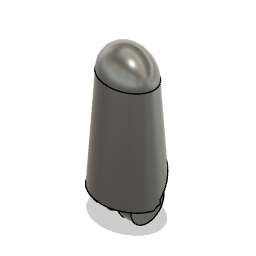
Bionic hand- flextion extention v2 (Autodesk Fusion 360 archive; units mm, degrees)
design "index part 1"
Autodesk Fusion 360 part; units mm, degrees
sketch "1st ellipse" plane through (0, 0, 0) normal (0, 1, 0) x (1, 0, 0)
  ellipse E0 centre (0, 0) end of major axis (5, 0) minor radius 4
  line L0 (-5, 0) -> (5, 0) construction
  line L1 (0, -4) -> (0, 4) construction
  constraint coincident E0 L0.start
  constraint coincident E0 L0.end
  constraint coincident E0 L1.start
  constraint coincident E0 L1.end
  constraint coincident E0.centre origin
  constraint horizontal L0
ref_plane "WorkPlane1" through (0, 15, 0) normal (0, 1, 0) x (1, 0, 0)
sketch "top elipse" plane through (0, 15, 0) normal (0, 1, 0) x (1, 0, 0)
  ellipse E0 centre (0, 0) end of major axis (4, 0) minor radius 3
  line L0 (-4, 0) -> (4, 0) construction
  line L1 (0, -3) -> (0, 3) construction
  constraint coincident E0 L0.start
  constraint coincident E0 L0.end
  constraint coincident E0 L1.start
  constraint coincident E0 L1.end
  constraint coincident E0.centre origin
  constraint horizontal L0
loft "Loft1" add profiles "1st ellipse", "top elipse" section 1 section 2 makes body 1
sketch "line over small elipse" plane through (0, 15, 0) normal (0, 1, 0) x (-1, 0, 0)
  ellipse E0 centre (0, 0) end of major axis (-4, 0) minor radius 3
  ellipse E1 centre (0, 0) end of major axis (-4, 0) minor radius 3
  line L0 (4, 0) -> (-4, 0) construction
  line L1 (0, 3) -> (0, -3) construction
  line L2 (0, -3) -> (0, 3)
  constraint coincident E1 L0.start
  constraint coincident E1 L0.end
  constraint coincident E1 L1.start
  constraint coincident E1 L1.end
  constraint coincident E0.centre E1.centre
  constraint horizontal L0
  constraint coincident L1.end L2.start
  constraint coincident L1.start L2.end
revolve "Revolve1" add sketch "line over small elipse" angle 360 about axis through (0, 15, 3) along (0, 0, -1) separate body contours E0 E1 L2 picked at (-0.4011, 0.9861) makes body 2
sketch "trapezium " plane through (0, 0, 0) normal (1, 0, 0) x (0, 0, -1)
  line L0 (0, 0) -> (0, 1)
  line L1 (0, 1) -> (4.5, 5.5)
  line L2 (4.5, 5.5) -> (4.5, 0)
  line L3 (4.5, 0) -> (0, 0)
  dimension "d3" = 1
  constraint coincident L0.start L3.end
  constraint vertical L0
  constraint parallel L0 L2
  constraint perpendicular L0 L3
  measures "d3" distance of L0.start L0.end
extrude "Extrude1" cut sketch "trapezium " along normal through all and the other way through all bodies 1
sketch "big circle" plane through (0, 0, 0) normal (1, 0, 0) x (0, 0, -1)
  circle A0 centre (0, -0.5) radius 2.5
  dimension "d5" = 5
  measures "d5" diameter of A0
extrude "Extrude2" add sketch "big circle" along normal mid plane 6 separate body makes body 3
extrude "Extrude3" cut 1 faces at (-3, -1.0437, -0.4573) along direction (1, 0, 0) blind 2 on bodies 3 bodies 1 3
extrude "Extrude4" cut 1 faces at (3, -1.0437, -0.4573) along direction (-1, 0, 0) blind 2 on bodies 3 bodies 1 3
sketch "small circle" plane through (-3, 0, 0) normal (1, 0, 0) x (0, 0, -1)
  line L0 (0, 1) -> (0.8508, 1.8508)
  arc A0 (0.8508, 1.8508) -> (-2.4495, 0) centre (0, -0.5) ccw
  line L1 (-2.4495, 0) -> (0, 0)
  line L2 (0, 0) -> (0, 1)
  circle A1 centre (0, -0.5) radius 1
  dimension "d12" = 2
  constraint concentric A0 A1
  measures "d12" diameter of A1
extrude "Extrude5" cut sketch "small circle" along normal mid plane 18 contours L1 L2 A1 | L1 L2 A1 bodies 1 3
sketch "Sketch7" plane through (0, 0, 0) normal (0, 0, 1) x (1, 0, 0)
sketch "Sketch8" plane through (0, 0, 0) normal (1, 0, 0) x (0, 0, -1)
extrude "Extrude6" add 1 faces at (1, -0.6739, -1.987) along direction (1, 0, 0) blind 2 on bodies 3 bodies 1 2 3
extrude "Extrude7" cut 1 faces at (-1, -2.4451, 0.4457) along direction (1, 0, 0) blind 2 on bodies 1 bodies 1
sketch "Sketch9" plane through (0, 0, 0) normal (1, 0, 0) x (0, 0, -1)
  circle A0 centre (0, -0.5) radius 2.5
  dimension "d19" = 5
  measures "d19" diameter of A0
extrude "Extrude8" add sketch "Sketch9" against normal blind 3 separate body makes body 4
extrude "Extrude9" cut 1 faces at (0, 0.1515, -0.5196) along direction (-1, 0, 0) blind 1 on bodies 4 bodies 4
extrude "Extrude10" cut sketch "small circle" along normal blind 3 contours L1 L2 A1 | L1 L2 A1 bodies 4

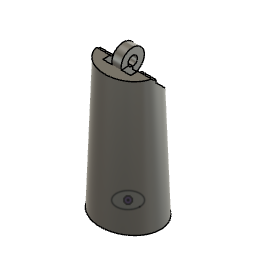
design "middle part 3"
Autodesk Fusion 360 part; units mm, degrees
sketch "Sketch1" plane through (0, 0, 0) normal (0, 1, 0) x (1, 0, 0)
  ellipse E0 centre (0, 0) end of major axis (7, 0) minor radius 6
  line L0 (-7, 0) -> (7, 0) construction
  line L1 (0, -6) -> (0, 6) construction
  dimension "d2" = 12
  constraint coincident E0 L0.start
  constraint coincident E0 L0.end
  constraint coincident E0 L1.start
  constraint coincident E0 L1.end
  constraint coincident E0.centre origin
  constraint horizontal L0
ref_plane "WorkPlane1" through (0, 28, 0) normal (0, 1, 0) x (1, 0, 0)
sketch "Sketch2" plane through (0, 28, 0) normal (0, 1, 0) x (1, 0, 0)
  ellipse E0 centre (0, 0) end of major axis (6, 0) minor radius 5
  line L0 (-6, 0) -> (6, 0) construction
  line L1 (0, -5) -> (0, 5) construction
  dimension "d3" = 10
  constraint coincident E0 L0.start
  constraint coincident E0 L0.end
  constraint coincident E0 L1.start
  constraint coincident E0 L1.end
  constraint coincident E0.centre origin
  constraint horizontal L0
sketch "Sketch3" plane through (0, 28, 0) normal (0, 1, 0) x (1, 0, 0)
loft "Loft1" add profiles "Sketch1", "Sketch2" section 1 section 2 makes body 1
sketch "Sketch4" plane through (0, 0, 0) normal (1, 0, 0) x (0, 0, -1)
  line L0 (0, 0) -> (0, 1)
  line L1 (7, 0) -> (0, 0)
  line L2 (0, 28) -> (0, 26.9237)
  line L3 (0, 26.9237) -> (5.6513, 21.2732)
  line L4 (5.6513, 21.2732) -> (5.6513, 28)
  line L5 (5.6513, 28) -> (0, 28)
  line L6 (0, 28) -> (0, 26.9237)
  line L7 (0, 28) -> (0, 26.9237)
  line L8 (0, 26.9237) -> (5.6513, 21.2732)
  line L9 (5.6513, 28) -> (0, 28)
  point P0 (0, 28)
  constraint coincident L0.start L1.end
  constraint vertical L0
  constraint perpendicular L0 L1
  constraint coincident P0 L2.start
  constraint vertical L2
  constraint parallel L2 L4
  constraint perpendicular L2 L5
  constraint coincident L2 L3.start
  constraint coincident L4 L3.end
extrude "Extrude1" cut sketch "Sketch4" along normal through all and the other way through all bodies 1
sketch "Sketch5" plane through (0, 0, 0) normal (1, 0, 0) x (0, 0, -1)
  circle A0 centre (0, -0.5) radius 2.5
  circle A1 centre (0, 28.5) radius 2.5
  dimension "d5" = 5
  dimension "d6" = 5
  measures "d5" diameter of A0
  measures "d6" diameter of A1
extrude "Extrude2" add sketch "Sketch5" along normal mid plane 6 separate body contours A1 makes body 2
extrude "Extrude3" cut 1 faces at (-3, 28.6214, -0.8056) along direction (1, 0, 0) blind 2 on bodies 2 bodies 1 2
extrude "Extrude4" cut 1 faces at (3, 28.6214, -0.8056) along direction (-1, 0, 0) blind 2 on bodies 2 bodies 1 2
sketch "Sketch6" plane through (0, 0, 0) normal (1, 0, 0) x (0, 0, -1)
  circle A0 centre (0, -0.5) radius 1
  circle A1 centre (0, 28.5) radius 1
  dimension "d15" = 2
  dimension "d16" = 2
  measures "d15" diameter of A0
  measures "d16" diameter of A1
extrude "Extrude6" cut sketch "Sketch6" along normal through all and the other way through all contours A1 bodies 1 2
ref_plane "WorkPlane2" through (0, 2, 0) normal (0, 1, 0) x (0, 0, 1)
sketch "Sketch7" plane through (0, 2, 0) normal (0, 1, 0) x (1, 0, 0)
  circle A0 centre (0, 0) radius 2.5
  dimension "d19" = 5
  constraint coincident A0.centre origin
  measures "d19" diameter of A0
sphere "SpherePrimitive1" cut diameter 5 placed x (1, 0, 0) y (0, 0, -1) z (0, 1, 0) at (0, 2, 0) bodies 1

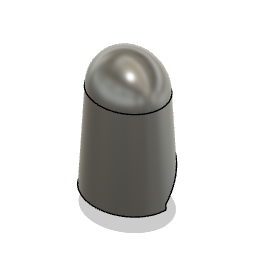
design "thumb part 1"
Autodesk Fusion 360 part; units mm, degrees
sketch "1st ellipse" plane through (0, 0, 0) normal (0, 1, 0) x (1, 0, 0)
  ellipse E0 centre (0, 0) end of major axis (8, 0) minor radius 7
  line L0 (-8, 0) -> (8, 0) construction
  line L1 (0, -7) -> (0, 7) construction
  ellipse E1 centre (0, 0) end of major axis (8, 0) minor radius 7
  line L2 (-8, 0) -> (8, 0) construction
  line L3 (0, -7) -> (0, 7) construction
  ellipse E2 centre (0, 0) end of major axis (8, 0) minor radius 7
  line L4 (-8, 0) -> (8, 0) construction
  line L5 (0, -7) -> (0, 7) construction
  constraint coincident E0 L0.start
  constraint coincident E0 L0.end
  constraint coincident E0 L1.start
  constraint coincident E0 L1.end
  constraint coincident E0.centre E1.centre
  constraint horizontal L0
  constraint coincident E1 L0.start
  constraint coincident E1 L0.end
  constraint coincident E1 L1.start
  constraint coincident E1 L1.end
  constraint concentric E0 E1
  constraint perpendicular L1 L2
  constraint coincident L1.end L3.end
  constraint coincident E2 L0.start
  constraint coincident E2 L0.end
  constraint coincident E2 L1.start
  constraint coincident E2 L1.end
  constraint concentric E0 E2
  constraint perpendicular L1 L4
  constraint coincident L0.end L2.end
ref_plane "WorkPlane1" through (0, 18, 0) normal (0, 1, 0) x (1, 0, 0)
sketch "top elipse" plane through (0, 18, 0) normal (0, 1, 0) x (1, 0, 0)
  ellipse E0 centre (0, 0) end of major axis (7, 0) minor radius 6
  line L0 (-7, 0) -> (7, 0) construction
  line L1 (0, -6) -> (0, 6) construction
  ellipse E1 centre (0, 0) end of major axis (7, 0) minor radius 6
  line L2 (-7, 0) -> (7, 0) construction
  line L3 (0, -6) -> (0, 6) construction
  dimension "d26" = 14
  dimension "d27" = 12
  dimension "d28" = 14
  constraint coincident E0 L0.start
  constraint coincident E0 L0.end
  constraint coincident E0 L1.start
  constraint coincident E0 L1.end
  constraint coincident E1 L0.start
  constraint coincident E1 L0.end
  constraint coincident E1 L1.start
  constraint coincident E1 L1.end
  constraint concentric E0 E1
  constraint coincident L1.end L3.end
  measures "d26" distance of E0
  measures "d28" distance of E1
loft "Loft1" add profiles "1st ellipse", "top elipse" section 1 section 2 makes body 1
sketch "line over small elipse" plane through (0, 18, 0) normal (0, 1, 0) x (-1, 0, 0)
  ellipse E0 centre (0, 0) end of major axis (-4, 0) minor radius 6
  line L0 (4, 0) -> (-4, 0) construction
  line L1 (0, 6) -> (0, -6) construction
  line L2 (0, -6) -> (0, 6)
  ellipse E1 centre (0, 0) end of major axis (-7, 0) minor radius 6
  constraint coincident E0 L0.start
  constraint coincident E0 L0.end
  constraint coincident E0 L1.start
  constraint coincident E0 L1.end
  constraint coincident E0.centre E1.centre
  constraint horizontal L0
  constraint coincident L1.end L2.start
  constraint coincident L1.start L2.end
  constraint coincident L1.start E1
revolve "Revolve1" add sketch "line over small elipse" angle 360 about axis through (0, 18, 6) along (0, 0, -1) separate body contours E0 E1 | E0 L2 picked at (-4.7303, 3.1798) picked at (-1.3308, 0.123) makes body 2
sketch "trapezium " plane through (0, 0, 0) normal (1, 0, 0) x (0, 0, -1)
  line L0 (0, 0) -> (0, 1)
  line L1 (0, 1) -> (9.6497, 10.621)
  line L2 (9.6497, 10.621) -> (9.6497, 0)
  line L3 (9.6497, 0) -> (0, 0)
  line L4 (0, 1) -> (9.648, 10.6193)
  line L5 (9.648, 10.6193) -> (9.648, 0)
  line L6 (9.648, 0) -> (0, 0)
  dimension "d3" = 1
  constraint coincident L0.start L3.end
  constraint vertical L0
  constraint parallel L0 L2
  constraint perpendicular L0 L3
  constraint parallel L1 L4
  constraint parallel L2 L5
  constraint perpendicular L0 L6
  measures "d3" distance of L0.start L0.end
extrude "Extrude1" cut sketch "trapezium " along normal through all and the other way through all bodies 1
sketch "big circle" plane through (0, 0, 0) normal (1, 0, 0) x (0, 0, -1)
  circle A0 centre (0, -0.5) radius 2.5
  dimension "d5" = 5
  measures "d5" diameter of A0
extrude "Extrude2" add sketch "big circle" along normal mid plane 6 separate body makes body 3
extrude "Extrude3" cut 1 faces at (-3, -1.0437, -0.4573) along direction (1, 0, 0) blind 2 on bodies 3 bodies 1 3
extrude "Extrude4" cut 1 faces at (3, -1.0437, -0.4573) along direction (-1, 0, 0) blind 2 on bodies 3 bodies 1 3
sketch "small circle" plane through (-3, 0, 0) normal (1, 0, 0) x (0, 0, -1)
  line L0 (0, 1) -> (0.8526, 1.8501)
  arc A0 (0.8526, 1.8501) -> (-2.4495, 0) centre (0, -0.5) ccw
  line L1 (-2.4495, 0) -> (0, 0)
  line L2 (0, 0) -> (0, 1)
  circle A1 centre (0, -0.5) radius 1
  dimension "d12" = 2
  constraint concentric A0 A1
  measures "d12" diameter of A1
extrude "Extrude5" cut sketch "small circle" along normal mid plane 18 contours L1 L2 A1 | L1 L2 A1 bodies 1 3
sketch "Sketch7" plane through (0, 0, 0) normal (0, 0, 1) x (1, 0, 0)
sketch "Sketch8" plane through (0, 0, 0) normal (1, 0, 0) x (0, 0, -1)
extrude "Extrude6" add 1 faces at (1, -0.6739, -1.987) along direction (1, 0, 0) blind 2 on bodies 3 bodies 1 2 3
extrude "Extrude7" cut 1 faces at (-1, -2.3582, 0.7275) along direction (1, 0, 0) blind 2 on bodies 1 bodies 1
sketch "Sketch9" plane through (0, 0, 0) normal (1, 0, 0) x (0, 0, -1)
  circle A0 centre (0, -0.5) radius 2.5
  dimension "d19" = 5
  measures "d19" diameter of A0
extrude "Extrude8" add sketch "Sketch9" against normal blind 3 separate body makes body 4
extrude "Extrude9" cut 1 faces at (0, 0.1515, -0.5196) along direction (-1, 0, 0) blind 1 on bodies 4 bodies 4
extrude "Extrude10" cut sketch "small circle" along normal blind 3 contours L1 L2 A1 | L1 L2 A1 bodies 4

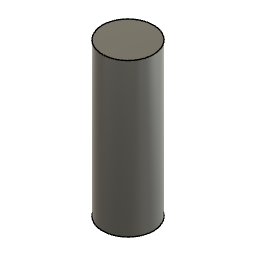
design "joint"
Autodesk Fusion 360 part; units mm, degrees
sketch "Sketch1" plane through (0, 0, 0) normal (0, 1, 0) x (1, 0, 0)
  circle A0 centre (0, 0) radius 1
  dimension "d1" = 2
  constraint coincident A0.centre origin
  measures "d1" diameter of A0
extrude "Extrude1" add sketch "Sketch1" along normal blind 6

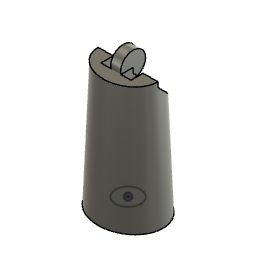
design "ring part 3"
Autodesk Fusion 360 part; units mm, degrees
sketch "Sketch1" plane through (0, 0, 0) normal (0, 1, 0) x (1, 0, 0)
  ellipse E0 centre (0, 0) end of major axis (7, 0) minor radius 6
  line L0 (-7, 0) -> (7, 0) construction
  line L1 (0, -6) -> (0, 6) construction
  dimension "d2" = 12
  constraint coincident E0 L0.start
  constraint coincident E0 L0.end
  constraint coincident E0 L1.start
  constraint coincident E0 L1.end
  constraint coincident E0.centre origin
  constraint horizontal L0
ref_plane "WorkPlane1" through (0, 25, 0) normal (0, 1, 0) x (1, 0, 0)
sketch "Sketch2" plane through (0, 25, 0) normal (0, 1, 0) x (1, 0, 0)
  ellipse E0 centre (0, 0) end of major axis (6, 0) minor radius 5
  line L0 (-6, 0) -> (6, 0) construction
  line L1 (0, -5) -> (0, 5) construction
  dimension "d3" = 10
  constraint coincident E0 L0.start
  constraint coincident E0 L0.end
  constraint coincident E0 L1.start
  constraint coincident E0 L1.end
  constraint coincident E0.centre origin
  constraint horizontal L0
sketch "Sketch3" plane through (0, 25, 0) normal (0, 1, 0) x (1, 0, 0)
loft "Loft1" add profiles "Sketch1", "Sketch2" section 1 section 2 makes body 1
sketch "Sketch4" plane through (0, 0, 0) normal (1, 0, 0) x (0, 0, -1)
  line L0 (0, 0) -> (0, 1)
  line L1 (0, 1) -> (7, 8)
  line L2 (7, 8) -> (7, 0)
  line L3 (7, 0) -> (0, 0)
  line L4 (0, 25) -> (0, 24)
  line L5 (0, 24) -> (5.5, 18.5)
  line L6 (5.5, 18.5) -> (5.5, 25)
  line L7 (5.5, 25) -> (0, 25)
  line L8 (0, 25) -> (0, 24)
  line L9 (0, 24) -> (5.5, 18.5027)
  line L10 (5.5, 25) -> (0, 25)
  point P0 (0, 25)
  constraint coincident L0.start L3.end
  constraint vertical L0
  constraint parallel L0 L2
  constraint perpendicular L0 L3
  constraint coincident P0 L4.start
  constraint vertical L4
  constraint parallel L4 L6
  constraint perpendicular L4 L7
  constraint coincident L4 L5.start
  constraint coincident L6 L9.end
extrude "Extrude1" cut sketch "Sketch4" along normal through all and the other way through all contours L4 L5 L6 L7 L8 L9 L10 bodies 1
sketch "Sketch5" plane through (0, 0, 0) normal (1, 0, 0) x (0, 0, -1)
  circle A0 centre (0, -0.5) radius 2.5
  circle A1 centre (0, 25.5) radius 2.5
  dimension "d5" = 5
  dimension "d6" = 5
  measures "d5" diameter of A0
  measures "d6" diameter of A1
extrude "Extrude2" add sketch "Sketch5" along normal mid plane 6 separate body contours A1 makes body 2
extrude "Extrude3" cut 1 faces at (-3, 25.6214, -0.8056) along direction (1, 0, 0) blind 2 on bodies 2 bodies 1 2
extrude "Extrude4" cut 1 faces at (3, 25.6214, -0.8056) along direction (-1, 0, 0) blind 2 on bodies 2 bodies 1 2
sketch "Sketch6" plane through (0, 0, 0) normal (1, 0, 0) x (0, 0, -1)
  circle A0 centre (0, 25.5) radius 1
  dimension "d16" = 2
  measures "d16" diameter of A0
ref_plane "WorkPlane2" through (0, 2, 0) normal (0, 1, 0) x (0, 0, 1)
sketch "Sketch7" plane through (0, 2, 0) normal (0, 1, 0) x (1, 0, 0)
  circle A0 centre (0, 0) radius 2.5
  dimension "d19" = 5
  constraint coincident A0.centre origin
  measures "d19" diameter of A0
sphere "SpherePrimitive1" cut diameter 5 placed x (1, 0, 0) y (0, 0, -1) z (0, 1, 0) at (0, 2, 0) bodies 1

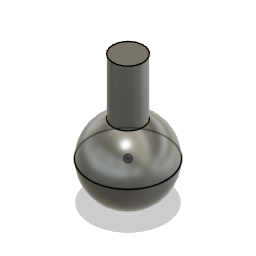
design "ball and socket joint"
Autodesk Fusion 360 part; units mm, degrees
sketch "Sketch1" plane through (0, 0, 0) normal (0, 1, 0) x (1, 0, 0)
  circle A0 centre (0, 0) radius 1
  dimension "d1" = 2
  constraint coincident A0.centre origin
  measures "d1" diameter of A0
extrude "Extrude1" add sketch "Sketch1" along normal blind 5 makes body 1
sketch "Sketch2" plane through (0, 0, 0) normal (0, 1, 0) x (1, 0, 0)
  circle A0 centre (0, 0) radius 2.5
  dimension "d4" = 5
  constraint coincident A0.centre origin
  measures "d4" diameter of A0
sphere "SpherePrimitive1" cut diameter 5.4 placed x (1, 0, 0) y (0, 0, -1) z (0, 1, 0) at (0, 0, 0) bodies 1
sphere "SpherePrimitive2" add diameter 5 placed x (1, 0, 0) y (0, 0, -1) z (0, 1, 0) at (0, 0, 0) separate body makes body 2
extrude "Extrude2" add 1 faces at (-0.3296, 5, -0.5031) along direction (0, -1, 0) blind 3 on bodies 1 bodies 1 2
extrude "Extrude3" add 1 faces at (-0.3296, 5, -0.5031) along direction (0, 1, 0) blind 1 on bodies 1 bodies 1

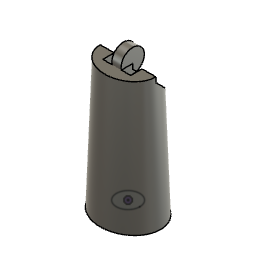
design "index part 3"
Autodesk Fusion 360 part; units mm, degrees
sketch "Sketch1" plane through (0, 0, 0) normal (0, 1, 0) x (1, 0, 0)
  ellipse E0 centre (0, 0) end of major axis (7, 0) minor radius 6
  line L0 (-7, 0) -> (7, 0) construction
  line L1 (0, -6) -> (0, 6) construction
  dimension "d2" = 12
  constraint coincident E0 L0.start
  constraint coincident E0 L0.end
  constraint coincident E0 L1.start
  constraint coincident E0 L1.end
  constraint coincident E0.centre origin
  constraint horizontal L0
ref_plane "WorkPlane1" through (0, 28, 0) normal (0, 1, 0) x (1, 0, 0)
sketch "Sketch2" plane through (0, 28, 0) normal (0, 1, 0) x (1, 0, 0)
  ellipse E0 centre (0, 0) end of major axis (6, 0) minor radius 5
  line L0 (-6, 0) -> (6, 0) construction
  line L1 (0, -5) -> (0, 5) construction
  dimension "d3" = 10
  constraint coincident E0 L0.start
  constraint coincident E0 L0.end
  constraint coincident E0 L1.start
  constraint coincident E0 L1.end
  constraint coincident E0.centre origin
  constraint horizontal L0
sketch "Sketch3" plane through (0, 28, 0) normal (0, 1, 0) x (1, 0, 0)
loft "Loft1" add profiles "Sketch1", "Sketch2" section 1 section 2 makes body 1
sketch "Sketch4" plane through (0, 0, 0) normal (1, 0, 0) x (0, 0, -1)
  line L0 (0, 0) -> (0, 1)
  line L1 (0, 1) -> (7, 8)
  line L2 (7, 8) -> (7, 0)
  line L3 (7, 0) -> (0, 0)
  line L4 (0, 28) -> (0, 26.9237)
  line L5 (0, 26.9237) -> (5.6513, 21.2732)
  line L6 (5.6513, 21.2732) -> (5.6513, 28)
  line L7 (5.6513, 28) -> (0, 28)
  line L8 (0, 28) -> (0, 26.9237)
  line L9 (0, 28) -> (0, 26.9237)
  line L10 (0, 26.9237) -> (5.6513, 21.2732)
  line L11 (5.6513, 28) -> (0, 28)
  point P0 (0, 28)
  constraint coincident L0.start L3.end
  constraint vertical L0
  constraint parallel L0 L2
  constraint perpendicular L0 L3
  constraint coincident P0 L4.start
  constraint vertical L4
  constraint parallel L4 L6
  constraint perpendicular L4 L7
  constraint coincident L4 L5.start
  constraint coincident L6 L5.end
extrude "Extrude1" cut sketch "Sketch4" along normal through all and the other way through all contours L4 L5 L6 L7 L8 L9 L10 L11 bodies 1
sketch "Sketch5" plane through (0, 0, 0) normal (1, 0, 0) x (0, 0, -1)
  circle A0 centre (0, -0.5) radius 2.5
  circle A1 centre (0, 28.5) radius 2.5
  dimension "d5" = 5
  dimension "d6" = 5
  measures "d5" diameter of A0
  measures "d6" diameter of A1
extrude "Extrude2" add sketch "Sketch5" along normal mid plane 6 separate body contours A1 makes body 2
extrude "Extrude3" cut 1 faces at (-3, 28.6214, -0.8056) along direction (1, 0, 0) blind 2 on bodies 2 bodies 1 2
extrude "Extrude4" cut 1 faces at (3, 28.6214, -0.8056) along direction (-1, 0, 0) blind 2 on bodies 2 bodies 1 2
sketch "Sketch6" plane through (0, 0, 0) normal (1, 0, 0) x (0, 0, -1)
  circle A0 centre (0, 28.5) radius 1
  dimension "d16" = 2
  measures "d16" diameter of A0
ref_plane "WorkPlane2" through (0, 2, 0) normal (0, 1, 0) x (0, 0, 1)
sketch "Sketch7" plane through (0, 2, 0) normal (0, 1, 0) x (1, 0, 0)
  circle A0 centre (0, 0) radius 2.5
  dimension "d19" = 5
  constraint coincident A0.centre origin
  measures "d19" diameter of A0
sphere "SpherePrimitive1" cut diameter 5 placed x (1, 0, 0) y (0, 0, -1) z (0, 1, 0) at (0, 2, 0) bodies 1

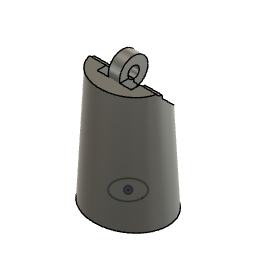
design "pinky part 3"
Autodesk Fusion 360 part; units mm, degrees
sketch "Sketch1" plane through (0, 0, 0) normal (0, 1, 0) x (1, 0, 0)
  ellipse E0 centre (0, 0) end of major axis (7, 0) minor radius 6
  line L0 (-7, 0) -> (7, 0) construction
  line L1 (0, -6) -> (0, 6) construction
  dimension "d2" = 12
  constraint coincident E0 L0.start
  constraint coincident E0 L0.end
  constraint coincident E0 L1.start
  constraint coincident E0 L1.end
  constraint coincident E0.centre origin
  constraint horizontal L0
ref_plane "WorkPlane1" through (0, 20, 0) normal (0, 1, 0) x (1, 0, 0)
sketch "Sketch2" plane through (0, 20, 0) normal (0, 1, 0) x (1, 0, 0)
  ellipse E0 centre (0, 0) end of major axis (6, 0) minor radius 5
  line L0 (-6, 0) -> (6, 0) construction
  line L1 (0, -5) -> (0, 5) construction
  dimension "d3" = 10
  constraint coincident E0 L0.start
  constraint coincident E0 L0.end
  constraint coincident E0 L1.start
  constraint coincident E0 L1.end
  constraint coincident E0.centre origin
  constraint horizontal L0
sketch "Sketch3" plane through (0, 20, 0) normal (0, 1, 0) x (1, 0, 0)
loft "Loft1" add profiles "Sketch1", "Sketch2" section 1 section 2 makes body 1
sketch "Sketch4" plane through (0, 0, 0) normal (1, 0, 0) x (0, 0, -1)
  line L0 (0, 0) -> (0, 1)
  line L1 (0, 20) -> (0, 19)
  line L2 (0, 19) -> (5.7581, 13.2325)
  line L3 (5.7581, 13.2325) -> (5.7581, 20)
  line L4 (5.7581, 20) -> (0, 20)
  point P0 (0, 20)
  dimension "d17" = 0
  constraint coincident L0.start origin
  constraint vertical L0
  constraint coincident P0 L1.start
  constraint vertical L1
  constraint parallel L1 L3
  constraint perpendicular L1 L4
extrude "Extrude1" cut sketch "Sketch4" along normal through all and the other way through all bodies 1
sketch "Sketch5" plane through (0, 0, 0) normal (1, 0, 0) x (0, 0, -1)
  circle A0 centre (0, -0.5) radius 2.5
  circle A1 centre (0, 20.5) radius 2.5
  dimension "d5" = 5
  dimension "d6" = 5
  measures "d5" diameter of A0
  measures "d6" diameter of A1
extrude "Extrude2" add sketch "Sketch5" along normal mid plane 6 separate body contours A1 makes body 2
extrude "Extrude3" cut 1 faces at (-3, 20.6214, -0.8056) along direction (1, 0, 0) blind 2 on bodies 2 bodies 1 2
extrude "Extrude4" cut 1 faces at (3, 20.6214, -0.8056) along direction (-1, 0, 0) blind 2 on bodies 2 bodies 1 2
sketch "Sketch6" plane through (0, 0, 0) normal (1, 0, 0) x (0, 0, -1)
  circle A0 centre (0, 20.5) radius 1
  dimension "d16" = 2
  measures "d16" diameter of A0
sketch "Sketch7" plane through (0, 0, 0) normal (1, 0, 0) x (0, 0, -1)
  circle A0 through (0.9826, 20.4973, -1) (-0.5174, 21.3634, -1) (-0.5174, 19.6313, -1)
  dimension "d18" = 2
extrude "Extrude7" cut sketch "Sketch7" along normal through all and the other way through all contours A0 in plane through (-1, 0, 0) normal (1, 0, 0) bodies 1 2
ref_plane "WorkPlane2" through (0, 2, 0) normal (0, 1, 0) x (0, 0, 1)
sketch "Sketch8" plane through (0, 2, 0) normal (0, 1, 0) x (1, 0, 0)
  circle A0 centre (0, 0) radius 2.5
  dimension "d21" = 5
  constraint coincident A0.centre origin
  measures "d21" diameter of A0
sphere "SpherePrimitive1" cut diameter 5 placed x (1, 0, 0) y (0, 0, -1) z (0, 1, 0) at (0, 2, 0) bodies 1

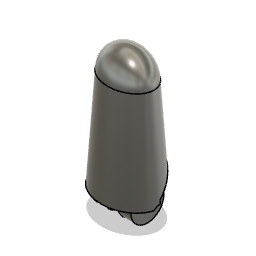
design "ring part 1"
Autodesk Fusion 360 part; units mm, degrees
sketch "1st ellipse" plane through (0, 0, 0) normal (0, 1, 0) x (1, 0, 0)
  ellipse E0 centre (0, 0) end of major axis (5, 0) minor radius 4
  line L0 (-5, 0) -> (5, 0) construction
  line L1 (0, -4) -> (0, 4) construction
  constraint coincident E0 L0.start
  constraint coincident E0 L0.end
  constraint coincident E0 L1.start
  constraint coincident E0 L1.end
  constraint coincident E0.centre origin
  constraint horizontal L0
ref_plane "WorkPlane1" through (0, 15, 0) normal (0, 1, 0) x (1, 0, 0)
sketch "top elipse" plane through (0, 15, 0) normal (0, 1, 0) x (1, 0, 0)
  ellipse E0 centre (0, 0) end of major axis (4, 0) minor radius 3
  line L0 (-4, 0) -> (4, 0) construction
  line L1 (0, -3) -> (0, 3) construction
  constraint coincident E0 L0.start
  constraint coincident E0 L0.end
  constraint coincident E0 L1.start
  constraint coincident E0 L1.end
  constraint coincident E0.centre origin
  constraint horizontal L0
loft "Loft1" add profiles "1st ellipse", "top elipse" section 1 section 2 makes body 1
sketch "line over small elipse" plane through (0, 15, 0) normal (0, 1, 0) x (-1, 0, 0)
  ellipse E0 centre (0, 0) end of major axis (-4, 0) minor radius 3
  ellipse E1 centre (0, 0) end of major axis (-4, 0) minor radius 3
  line L0 (4, 0) -> (-4, 0) construction
  line L1 (0, 3) -> (0, -3) construction
  line L2 (0, -3) -> (0, 3)
  constraint coincident E1 L0.start
  constraint coincident E1 L0.end
  constraint coincident E1 L1.start
  constraint coincident E1 L1.end
  constraint coincident E0.centre E1.centre
  constraint horizontal L0
  constraint coincident L1.end L2.start
  constraint coincident L1.start L2.end
revolve "Revolve1" add sketch "line over small elipse" angle 360 about axis through (0, 15, 3) along (0, 0, -1) separate body contours E0 E1 L2 picked at (-0.4011, 0.9861) makes body 2
sketch "trapezium " plane through (0, 0, 0) normal (1, 0, 0) x (0, 0, -1)
  line L0 (0, 0) -> (0, 1)
  line L1 (0, 1) -> (4.5, 5.5)
  line L2 (4.5, 5.5) -> (4.5, 0)
  line L3 (4.5, 0) -> (0, 0)
  dimension "d3" = 1
  constraint coincident L0.start L3.end
  constraint vertical L0
  constraint parallel L0 L2
  constraint perpendicular L0 L3
  measures "d3" distance of L0.start L0.end
extrude "Extrude1" cut sketch "trapezium " along normal through all and the other way through all bodies 1
sketch "big circle" plane through (0, 0, 0) normal (1, 0, 0) x (0, 0, -1)
  circle A0 centre (0, -0.5) radius 2.5
  dimension "d5" = 5
  measures "d5" diameter of A0
extrude "Extrude2" add sketch "big circle" along normal mid plane 6 separate body makes body 3
extrude "Extrude3" cut 1 faces at (-3, -1.0437, -0.4573) along direction (1, 0, 0) blind 2 on bodies 3 bodies 1 3
extrude "Extrude4" cut 1 faces at (3, -1.0437, -0.4573) along direction (-1, 0, 0) blind 2 on bodies 3 bodies 1 3
sketch "small circle" plane through (-3, 0, 0) normal (1, 0, 0) x (0, 0, -1)
  line L0 (0, 1) -> (0.8508, 1.8508)
  arc A0 (0.8508, 1.8508) -> (-2.4495, 0) centre (0, -0.5) ccw
  line L1 (-2.4495, 0) -> (0, 0)
  line L2 (0, 0) -> (0, 1)
  circle A1 centre (0, -0.5) radius 1
  dimension "d12" = 2
  constraint concentric A0 A1
  measures "d12" diameter of A1
extrude "Extrude5" cut sketch "small circle" along normal mid plane 18 contours L1 L2 A1 | L1 L2 A1 bodies 1 3
sketch "Sketch7" plane through (0, 0, 0) normal (0, 0, 1) x (1, 0, 0)
sketch "Sketch8" plane through (0, 0, 0) normal (1, 0, 0) x (0, 0, -1)
extrude "Extrude6" add 1 faces at (1, -0.6739, -1.987) along direction (1, 0, 0) blind 2 on bodies 3 bodies 1 2 3
extrude "Extrude7" cut 1 faces at (-1, -2.4451, 0.4457) along direction (1, 0, 0) blind 2 on bodies 1 bodies 1
sketch "Sketch9" plane through (0, 0, 0) normal (1, 0, 0) x (0, 0, -1)
  circle A0 centre (0, -0.5) radius 2.5
  dimension "d19" = 5
  measures "d19" diameter of A0
extrude "Extrude8" add sketch "Sketch9" against normal blind 3 separate body makes body 4
extrude "Extrude9" cut 1 faces at (0, 0.1515, -0.5196) along direction (-1, 0, 0) blind 1 on bodies 4 bodies 4
extrude "Extrude10" cut sketch "small circle" along normal blind 3 contours L1 L2 A1 | L1 L2 A1 bodies 4

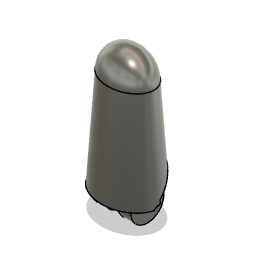
design "pinky part 1"
Autodesk Fusion 360 part; units mm, degrees
sketch "1st ellipse" plane through (0, 0, 0) normal (0, 1, 0) x (1, 0, 0)
  ellipse E0 centre (0, 0) end of major axis (5, 0) minor radius 4
  line L0 (-5, 0) -> (5, 0) construction
  line L1 (0, -4) -> (0, 4) construction
  constraint coincident E0 L0.start
  constraint coincident E0 L0.end
  constraint coincident E0 L1.start
  constraint coincident E0 L1.end
  constraint coincident E0.centre origin
  constraint horizontal L0
ref_plane "WorkPlane1" through (0, 15, 0) normal (0, 1, 0) x (1, 0, 0)
sketch "top elipse" plane through (0, 15, 0) normal (0, 1, 0) x (1, 0, 0)
  ellipse E0 centre (0, 0) end of major axis (4, 0) minor radius 3
  line L0 (-4, 0) -> (4, 0) construction
  line L1 (0, -3) -> (0, 3) construction
  constraint coincident E0 L0.start
  constraint coincident E0 L0.end
  constraint coincident E0 L1.start
  constraint coincident E0 L1.end
  constraint coincident E0.centre origin
  constraint horizontal L0
loft "Loft1" add profiles "1st ellipse", "top elipse" section 1 section 2 makes body 1
sketch "line over small elipse" plane through (0, 15, 0) normal (0, 1, 0) x (-1, 0, 0)
  ellipse E0 centre (0, 0) end of major axis (-4, 0) minor radius 3
  ellipse E1 centre (0, 0) end of major axis (-4, 0) minor radius 3
  line L0 (4, 0) -> (-4, 0) construction
  line L1 (0, 3) -> (0, -3) construction
  line L2 (0, -3) -> (0, 3)
  constraint coincident E1 L0.start
  constraint coincident E1 L0.end
  constraint coincident E1 L1.start
  constraint coincident E1 L1.end
  constraint coincident E0.centre E1.centre
  constraint horizontal L0
  constraint coincident L1.end L2.start
  constraint coincident L1.start L2.end
revolve "Revolve1" add sketch "line over small elipse" angle 360 about axis through (0, 15, 3) along (0, 0, -1) separate body contours E0 E1 L2 picked at (-0.4011, 0.9861) makes body 2
sketch "trapezium " plane through (0, 0, 0) normal (1, 0, 0) x (0, 0, -1)
  line L0 (0, 0) -> (0, 1)
  line L1 (0, 1) -> (4.5, 5.5)
  line L2 (4.5, 5.5) -> (4.5, 0)
  line L3 (4.5, 0) -> (0, 0)
  dimension "d3" = 1
  constraint coincident L0.start L3.end
  constraint vertical L0
  constraint parallel L0 L2
  constraint perpendicular L0 L3
  measures "d3" distance of L0.start L0.end
extrude "Extrude1" cut sketch "trapezium " along normal through all and the other way through all bodies 1
sketch "big circle" plane through (0, 0, 0) normal (1, 0, 0) x (0, 0, -1)
  circle A0 centre (0, -0.5) radius 2.5
  dimension "d5" = 5
  measures "d5" diameter of A0
extrude "Extrude2" add sketch "big circle" along normal mid plane 6 separate body makes body 3
extrude "Extrude3" cut 1 faces at (-3, -1.0437, -0.4573) along direction (1, 0, 0) blind 2 on bodies 3 bodies 1 3
extrude "Extrude4" cut 1 faces at (3, -1.0437, -0.4573) along direction (-1, 0, 0) blind 2 on bodies 3 bodies 1 3
sketch "small circle" plane through (-3, 0, 0) normal (1, 0, 0) x (0, 0, -1)
  line L0 (0, 1) -> (0.8508, 1.8508)
  arc A0 (0.8508, 1.8508) -> (-2.4495, 0) centre (0, -0.5) ccw
  line L1 (-2.4495, 0) -> (0, 0)
  line L2 (0, 0) -> (0, 1)
  circle A1 centre (0, -0.5) radius 1
  dimension "d12" = 2
  constraint concentric A0 A1
  measures "d12" diameter of A1
extrude "Extrude5" cut sketch "small circle" along normal mid plane 18 contours L1 L2 A1 | L1 L2 A1 bodies 1 3
sketch "Sketch7" plane through (0, 0, 0) normal (0, 0, 1) x (1, 0, 0)
sketch "Sketch8" plane through (0, 0, 0) normal (1, 0, 0) x (0, 0, -1)
extrude "Extrude6" add 1 faces at (1, -0.6739, -1.987) along direction (1, 0, 0) blind 2 on bodies 3 bodies 1 2 3
extrude "Extrude7" cut 1 faces at (-1, -2.4451, 0.4457) along direction (1, 0, 0) blind 2 on bodies 1 bodies 1
sketch "Sketch9" plane through (0, 0, 0) normal (1, 0, 0) x (0, 0, -1)
  circle A0 centre (0, -0.5) radius 2.5
  dimension "d19" = 5
  measures "d19" diameter of A0
extrude "Extrude8" add sketch "Sketch9" against normal blind 3 separate body makes body 4
extrude "Extrude9" cut 1 faces at (0, 0.1515, -0.5196) along direction (-1, 0, 0) blind 1 on bodies 4 bodies 4
extrude "Extrude10" cut sketch "small circle" along normal blind 3 contours L1 L2 A1 | L1 L2 A1 bodies 4

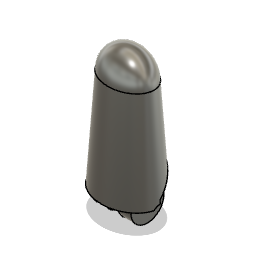
design "middle part 1"
Autodesk Fusion 360 part; units mm, degrees
sketch "1st ellipse" plane through (0, 0, 0) normal (0, 1, 0) x (1, 0, 0)
  ellipse E0 centre (0, 0) end of major axis (5, 0) minor radius 4
  line L0 (-5, 0) -> (5, 0) construction
  line L1 (0, -4) -> (0, 4) construction
  constraint coincident E0 L0.start
  constraint coincident E0 L0.end
  constraint coincident E0 L1.start
  constraint coincident E0 L1.end
  constraint coincident E0.centre origin
  constraint horizontal L0
ref_plane "WorkPlane1" through (0, 15, 0) normal (0, 1, 0) x (1, 0, 0)
sketch "top elipse" plane through (0, 15, 0) normal (0, 1, 0) x (1, 0, 0)
  ellipse E0 centre (0, 0) end of major axis (4, 0) minor radius 3
  line L0 (-4, 0) -> (4, 0) construction
  line L1 (0, -3) -> (0, 3) construction
  constraint coincident E0 L0.start
  constraint coincident E0 L0.end
  constraint coincident E0 L1.start
  constraint coincident E0 L1.end
  constraint coincident E0.centre origin
  constraint horizontal L0
loft "Loft1" add profiles "1st ellipse", "top elipse" section 1 section 2 makes body 1
sketch "line over small elipse" plane through (0, 15, 0) normal (0, 1, 0) x (-1, 0, 0)
  ellipse E0 centre (0, 0) end of major axis (-4, 0) minor radius 3
  ellipse E1 centre (0, 0) end of major axis (-4, 0) minor radius 3
  line L0 (4, 0) -> (-4, 0) construction
  line L1 (0, 3) -> (0, -3) construction
  line L2 (0, -3) -> (0, 3)
  constraint coincident E1 L0.start
  constraint coincident E1 L0.end
  constraint coincident E1 L1.start
  constraint coincident E1 L1.end
  constraint coincident E0.centre E1.centre
  constraint horizontal L0
  constraint coincident L1.end L2.start
  constraint coincident L1.start L2.end
revolve "Revolve1" add sketch "line over small elipse" angle 360 about axis through (0, 15, 3) along (0, 0, -1) separate body contours E0 E1 L2 picked at (-0.4011, 0.9861) makes body 2
sketch "trapezium " plane through (0, 0, 0) normal (1, 0, 0) x (0, 0, -1)
  line L0 (0, 0) -> (0, 1)
  line L1 (0, 1) -> (4.5, 5.5)
  line L2 (4.5, 5.5) -> (4.5, 0)
  line L3 (4.5, 0) -> (0, 0)
  dimension "d3" = 1
  constraint coincident L0.start L3.end
  constraint vertical L0
  constraint parallel L0 L2
  constraint perpendicular L0 L3
  measures "d3" distance of L0.start L0.end
extrude "Extrude1" cut sketch "trapezium " along normal through all and the other way through all bodies 1
sketch "big circle" plane through (0, 0, 0) normal (1, 0, 0) x (0, 0, -1)
  circle A0 centre (0, -0.5) radius 2.5
  dimension "d5" = 5
  measures "d5" diameter of A0
extrude "Extrude2" add sketch "big circle" along normal mid plane 6 separate body makes body 3
extrude "Extrude3" cut 1 faces at (-3, -1.0437, -0.4573) along direction (1, 0, 0) blind 2 on bodies 3 bodies 1 3
extrude "Extrude4" cut 1 faces at (3, -1.0437, -0.4573) along direction (-1, 0, 0) blind 2 on bodies 3 bodies 1 3
sketch "small circle" plane through (-3, 0, 0) normal (1, 0, 0) x (0, 0, -1)
  line L0 (0, 1) -> (0.8508, 1.8508)
  arc A0 (0.8508, 1.8508) -> (-2.4495, 0) centre (0, -0.5) ccw
  line L1 (-2.4495, 0) -> (0, 0)
  line L2 (0, 0) -> (0, 1)
  circle A1 centre (0, -0.5) radius 1
  dimension "d12" = 2
  constraint concentric A0 A1
  measures "d12" diameter of A1
extrude "Extrude5" cut sketch "small circle" along normal mid plane 18 contours L1 L2 A1 | L1 L2 A1 bodies 1 3
sketch "Sketch7" plane through (0, 0, 0) normal (0, 0, 1) x (1, 0, 0)
sketch "Sketch8" plane through (0, 0, 0) normal (1, 0, 0) x (0, 0, -1)
extrude "Extrude6" add 1 faces at (1, -0.6739, -1.987) along direction (1, 0, 0) blind 2 on bodies 3 bodies 1 2 3
extrude "Extrude7" cut 1 faces at (-1, -2.4451, 0.4457) along direction (1, 0, 0) blind 2 on bodies 1 bodies 1
sketch "Sketch9" plane through (0, 0, 0) normal (1, 0, 0) x (0, 0, -1)
  circle A0 centre (0, -0.5) radius 2.5
  dimension "d19" = 5
  measures "d19" diameter of A0
extrude "Extrude8" add sketch "Sketch9" against normal blind 3 separate body makes body 4
extrude "Extrude9" cut 1 faces at (0, 0.1515, -0.5196) along direction (-1, 0, 0) blind 1 on bodies 4 bodies 4
extrude "Extrude10" cut sketch "small circle" along normal blind 3 contours L1 L2 A1 | L1 L2 A1 bodies 4
